Autodesk Fusion 360 part; units mm, degrees
(part 2 of 3)
sketch "Sketch7" plane through (0, 0, 3) normal (0, 0, 1) x (-1, 0, 0)
  line L0 (35, -173) -> (35, -178)
  line L1 (35, -178) -> (-35, -178)
  line L2 (-35, -178) -> (-35, -173)
  line L3 (-35, -173) -> (35, -173)
  line L4 (-35, -238) -> (-35, -233)
  line L5 (-35, -233) -> (35, -233)
  line L6 (35, -233) -> (35, -238)
  line L7 (35, -238) -> (-35, -238)
  circle A0 centre (-24.25, -133) radius 1.5
  circle A1 centre (24.25, -71.5) radius 1.5
  circle A2 centre (24.25, -133) radius 1.5
  circle A3 centre (-24.25, -71.5) radius 1.5
  line L8 (46.5, -10) -> (46.5, -15)
  line L9 (46.5, -15) -> (-46.5, -15)
  line L10 (-46.5, -15) -> (-46.5, -10)
  line L11 (-46.5, -10) -> (46.5, -10)
  line L12 (-46.5, -63) -> (-46.5, -58)
  line L13 (-46.5, -58) -> (46.5, -58)
  line L14 (46.5, -58) -> (46.5, -63)
  line L15 (46.5, -63) -> (-46.5, -63)
  line L16 (51.5, 0) -> (-51.5, 0)
  line L17 (-51.5, 0) -> (-51.5, -265)
  line L18 (-51.5, -265) -> (51.5, -265)
  line L19 (51.5, -265) -> (51.5, 0)
  line L20 (0, -238) -> (0, -248)
  line L21 (0, -248) -> (3, -248)
  line L22 (0, -248) -> (-3, -248)
  line L23 (0, -265) -> (0, -260)
  line L24 (3, -248) -> (3, -258)
  line L25 (3, -258) -> (8, -258)
  line L26 (3, -248) -> (8, -248)
  line L27 (8, -258) -> (8, -248)
  line L28 (-3, -248) -> (-3, -258)
  line L29 (-3, -258) -> (-8, -258)
  line L30 (-8, -258) -> (-8, -248)
  line L31 (-3, -248) -> (-8, -248)
  dimension "d38" = 10
  dimension "d39" = 3
  dimension "d40" = 3
  dimension "d41" = 5
  dimension "d42" = 10
  dimension "d43" = 5
  dimension "d44" = 5
  dimension "d45" = 5
  dimension "d46" = 10
  constraint midpoint L7 L20.start
  constraint perpendicular L7 L20
  constraint perpendicular L20 L21
  constraint perpendicular L20 L22
  constraint midpoint L18 L23.start
  constraint perpendicular L18 L23
  constraint perpendicular L21 L24
  constraint perpendicular L24 L25
  constraint perpendicular L20 L26
  constraint perpendicular L22 L28
  constraint perpendicular L28 L29
  constraint perpendicular L29 L30
  constraint perpendicular L30 L31
  measures "d38" distance of L20.start L20.end
  measures "d39" distance of L20.end L21.end
  measures "d40" distance of L20.end L22.end
  measures "d41" distance of L23.start L23.end
  measures "d42" distance of L21.end L24.end
  measures "d43" distance of L24.end L25.end
  measures "d44" distance of L21.end L26.end
  measures "d45" distance of L28.end L29.end
  measures "d46" distance of L29.end L30.end
extrude "Extrude7" add sketch "Sketch7" along normal blind 6 contours L24 L25 L26 L27 | L28 L29 L30 L31
sketch "Sketch8" plane through (8, 0, 0) normal (1, 0, 0) x (0, 1, 0)
  line L0 (248, 3) -> (258, 3)
  line L1 (258, 3) -> (258, 9)
  line L2 (258, 9) -> (248, 9)
  line L3 (248, 9) -> (248, 3)
  line L4 (253, 3) -> (253, 9)
  circle A0 centre (253, 6) radius 1.5
  dimension "d49" = 3
  constraint midpoint L0 L4.start
  constraint midpoint L2 L4.end
  constraint midpoint L4 A0.centre
  measures "d49" diameter of A0
extrude "Extrude8" cut sketch "Sketch8" against normal blind 20 contours L4 A0 | L4 A0
fillet "Fillet1" radius 10 4 edges at (51.5, 0, 1.5) (-51.5, 0, 1.5) (51.5, 265, 1.5) (-51.5, 265, 1.5)
fillet "Fillet2" radius 5 8 edges at (51.5, 132.5, 0) (48.5711, 262.0711, 0) (0, 265, 0) (-48.5711, 262.0711, 0) (-51.5, 132.5, 0) (-48.5711, 2.9289, 0) (0, 0, 0) (48.5711, 2.9289, 0)
sketch "Sketch9" plane through (0, 0, 3) normal (0, 0, 1) x (-1, 0, 0)
  arc A0 (41.5, -265) -> (51.5, -255) centre (41.5, -255) ccw
  line L0 (51.5, -255) -> (51.5, -10)
  arc A1 (51.5, -10) -> (41.5, 0) centre (41.5, -10) ccw
  line L1 (41.5, 0) -> (-41.5, 0)
  arc A2 (-41.5, 0) -> (-51.5, -10) centre (-41.5, -10) ccw
  line L2 (-51.5, -10) -> (-51.5, -255)
  arc A3 (-51.5, -255) -> (-41.5, -265) centre (-41.5, -255) ccw
  line L3 (-41.5, -265) -> (41.5, -265)
  line L4 (-3, -258) -> (-8, -258)
  line L5 (-8, -258) -> (-8, -248)
  line L6 (-8, -248) -> (-3, -248)
  line L7 (-3, -248) -> (-3, -258)
  line L8 (3, -248) -> (8, -248)
  line L9 (8, -248) -> (8, -258)
  line L10 (8, -258) -> (3, -258)
  line L11 (3, -258) -> (3, -248)
  line L12 (35, -173) -> (35, -178)
  line L13 (35, -178) -> (-35, -178)
  line L14 (-35, -178) -> (-35, -173)
  line L15 (-35, -173) -> (35, -173)
  line L16 (-35, -238) -> (-35, -233)
  line L17 (-35, -233) -> (35, -233)
  line L18 (35, -233) -> (35, -238)
  line L19 (35, -238) -> (-35, -238)
  circle A4 centre (-24.25, -133) radius 1.5
  circle A5 centre (24.25, -71.5) radius 1.5
  circle A6 centre (24.25, -133) radius 1.5
  circle A7 centre (-24.25, -71.5) radius 1.5
  line L20 (46.5, -10) -> (46.5, -15)
  line L21 (46.5, -15) -> (-46.5, -15)
  line L22 (-46.5, -15) -> (-46.5, -10)
  line L23 (-46.5, -10) -> (46.5, -10)
  line L24 (-46.5, -63) -> (-46.5, -58)
  line L25 (-46.5, -58) -> (46.5, -58)
  line L26 (46.5, -58) -> (46.5, -63)
  line L27 (46.5, -63) -> (-46.5, -63)
  line L28 (0, -58) -> (0, -15)
  line L29 (0, -36.5) -> (20, -36.5)
  line L30 (0, -36.5) -> (-20, -36.5)
  line L31 (20, -36.5) -> (20, -46.5)
  line L32 (-20, -36.5) -> (-20, -46.5)
  line L33 (20, -46.5) -> (-20, -46.5)
  line L34 (20, -36.5) -> (20, -26.5)
  line L35 (20, -26.5) -> (-20, -26.5)
  line L36 (-20, -36.5) -> (-20, -26.5)
  dimension "d56" = 20
  dimension "d57" = 20
  dimension "d58" = 10
  dimension "d59" = 10
  dimension "d60" = 10
  dimension "d61" = 40
  constraint midpoint L25 L28.start
  constraint midpoint L21 L28.end
  constraint midpoint L28 L29.start
  constraint perpendicular L28 L29
  constraint perpendicular L28 L30
  constraint perpendicular L25 L31
  constraint perpendicular L30 L32
  constraint perpendicular L29 L34
  constraint perpendicular L28 L35
  measures "d56" distance of L29.start L29.end
  measures "d57" distance of L29.start L30.end
  measures "d58" distance of L29.end L31.end
  measures "d59" distance of L30.end L32.end
  measures "d60" distance of L29.end L34.end
  measures "d61" distance of L34.end L35.end
extrude "Extrude9" cut sketch "Sketch9" against normal blind 5 contours L28 L30 L32 L33 | L28 L29 L31 L33 | L28 L30 L35 L36 | L28 L29 L34 L35
sketch "Sketch10" plane through (0, 0, 9) normal (0, 0, 1) x (-1, 0, 0)
  line L0 (-46.5, -63) -> (46.5, -63)
  line L1 (46.5, -63) -> (46.5, -58)
  line L2 (46.5, -58) -> (-46.5, -58)
  line L3 (-46.5, -58) -> (-46.5, -63)
  line L4 (46.5, -60.5) -> (28.5, -60.5)
  circle A0 centre (28.5, -60.5) radius 1.5
  line L5 (0, -58) -> (0, -50)
  line L6 (46.5, -58) -> (46.5, -15)
  line L7 (46.5, -36.5) -> (70, -36.5)
  circle A1 centre (28.5, -12.5) radius 1.5
  circle A2 centre (-28.5, -60.5) radius 1.5
  circle A3 centre (-28.5, -12.5) radius 1.5
  point P0 (28.5, -12.5)
  dimension "d64" = 18
  dimension "d65" = 3
  dimension "d66" = 3
  constraint midpoint L1 L4.start
  constraint perpendicular L1 L4
  constraint coincident L4.end A0.centre
  constraint midpoint L2 L5.start
  constraint perpendicular L2 L5
  constraint coincident L1.end L2.start
  constraint perpendicular L2 L6
  constraint midpoint L6 L7.start
  constraint perpendicular L6 L7
  constraint symmetric L4.end L7 P0
  constraint coincident P0 A1.centre
  constraint symmetric A0 L5 A2
  constraint symmetric L5 A1 A3
  measures "d64" distance of L4.start L4.end
  measures "d65" diameter of A0
  measures "d66" diameter of A1
extrude "Extrude10" cut sketch "Sketch10" against normal blind 50 contours A0 | A1 | A2 | A3
sketch "Sketch11" plane through (0, 0, 3) normal (0, 0, 1) x (-1, 0, 0)
  line L0 (-20, -26.5) -> (20, -26.5)
  line L1 (20, -26.5) -> (20, -46.5)
  line L2 (20, -46.5) -> (-20, -46.5)
  line L3 (-20, -46.5) -> (-20, -26.5)
  arc A0 (41.5, -265) -> (51.5, -255) centre (41.5, -255) ccw
  line L4 (51.5, -255) -> (51.5, -10)
  arc A1 (51.5, -10) -> (41.5, 0) centre (41.5, -10) ccw
  line L5 (41.5, 0) -> (-41.5, 0)
  arc A2 (-41.5, 0) -> (-51.5, -10) centre (-41.5, -10) ccw
  line L6 (-51.5, -10) -> (-51.5, -255)
  arc A3 (-51.5, -255) -> (-41.5, -265) centre (-41.5, -255) ccw
  line L7 (-41.5, -265) -> (41.5, -265)
  line L8 (-3, -258) -> (-8, -258)
  line L9 (-8, -258) -> (-8, -248)
  line L10 (-8, -248) -> (-3, -248)
  line L11 (-3, -248) -> (-3, -258)
  line L12 (3, -248) -> (8, -248)
  line L13 (8, -248) -> (8, -258)
  line L14 (8, -258) -> (3, -258)
  line L15 (3, -258) -> (3, -248)
  line L16 (35, -173) -> (35, -178)
  line L17 (35, -178) -> (-35, -178)
  line L18 (-35, -178) -> (-35, -173)
  line L19 (-35, -173) -> (35, -173)
  line L20 (-35, -238) -> (-35, -233)
  line L21 (-35, -233) -> (35, -233)
  line L22 (35, -233) -> (35, -238)
  line L23 (35, -238) -> (-35, -238)
  circle A4 centre (-24.25, -133) radius 1.5
  circle A5 centre (24.25, -71.5) radius 1.5
  circle A6 centre (24.25, -133) radius 1.5
  circle A7 centre (-24.25, -71.5) radius 1.5
  line L24 (46.5, -10) -> (46.5, -15)
  line L25 (46.5, -15) -> (-46.5, -15)
  line L26 (-46.5, -15) -> (-46.5, -10)
  line L27 (-46.5, -10) -> (46.5, -10)
  line L28 (-46.5, -63) -> (-46.5, -58)
  line L29 (-46.5, -58) -> (46.5, -58)
  line L30 (46.5, -58) -> (46.5, -63)
  line L31 (46.5, -63) -> (-46.5, -63)
  line L32 (51.5, -255) -> (48.5, -255)
  circle A8 centre (48.5, -255) radius 1.5
  line L33 (51.5, -132.5) -> (48.5, -132.5)
  circle A9 centre (48.5, -132.5) radius 1.5
  line L34 (48.5, -255) -> (48.5, -132.5)
  circle A10 centre (48.5, -193.75) radius 1.5
  line L35 (0, -265) -> (0, -262)
  circle A11 centre (0, -262) radius 1.5
  circle A12 centre (0, -3) radius 1.5
  circle A13 centre (48.5, -10) radius 1.5
  circle A14 centre (48.5, -71.25) radius 1.5
  circle A15 centre (48.5, -132.5) radius 1.5
  circle A16 centre (-48.5, -10) radius 1.5
  circle A17 centre (-48.5, -71.25) radius 1.5
  circle A18 centre (-48.5, -132.5) radius 1.5
  circle A19 centre (-48.5, -193.75) radius 1.5
  circle A20 centre (-48.5, -255) radius 1.5
  dimension "d69" = 3
  dimension "d70" = 3
  dimension "d71" = 3
  dimension "d72" = 3
  dimension "d73" = 3
  dimension "d74" = 3
  dimension "d75" = 3
  constraint coincident A0.end L4.start
  constraint perpendicular L4 L32
  constraint coincident L32.end A8.centre
  constraint midpoint L4 L33.start
  constraint perpendicular L4 L33
  constraint coincident L33.end A9.centre
  constraint midpoint L34 A10.centre
  constraint midpoint L7 L35.start
  constraint perpendicular L7 L35
  constraint coincident L35.end A11.centre
  constraint symmetric A8 L33 A13
  constraint symmetric L33 A9 A15
  constraint symmetric L33 A10 A14
  constraint symmetric L33 A11 A12
  constraint symmetric A8 L35 A20
  constraint symmetric A10 L35 A19
  constraint symmetric L35 A13 A16
  constraint symmetric L35 A14 A17
  constraint symmetric L35 A15 A18
  measures "d69" distance of A0.end L32.end
  measures "d70" diameter of A8
  measures "d71" distance of L33.start L33.end
  measures "d72" diameter of A9
  measures "d73" diameter of A10
  measures "d74" distance of L35.start L35.end
  measures "d75" diameter of A11
extrude "Extrude11" cut sketch "Sketch11" against normal blind 5 contours L32 A8 L34 | L32 A8 L34 | L33 A9 L34 A15 | L33 A9 L34 A15 | L34 A10 | L34 A10 | A11 | A12 | A13 | A14 | A16 | A17 | A18 | A19 | A20
sketch "Sketch12" plane through (0, 0, 3) normal (0, 0, 1) x (-1, 0, 0)
  circle A0 centre (48.5, -255) radius 1.5
  circle A1 centre (-48.5, -193.75) radius 1.5
  circle A2 centre (-48.5, -10) radius 1.5
  circle A3 centre (48.5, -10) radius 1.5
  circle A4 centre (-48.5, -132.5) radius 1.5
  circle A5 centre (0, -262) radius 1.5
  circle A6 centre (48.5, -193.75) radius 1.5
  circle A7 centre (-48.5, -71.25) radius 1.5
  circle A8 centre (0, -3) radius 1.5
  circle A9 centre (48.5, -71.25) radius 1.5
  circle A10 centre (48.5, -132.5) radius 1.5
  circle A11 centre (-48.5, -255) radius 1.5
  line L0 (-20, -26.5) -> (20, -26.5)
  line L1 (20, -26.5) -> (20, -46.5)
  line L2 (20, -46.5) -> (-20, -46.5)
  line L3 (-20, -46.5) -> (-20, -26.5)
  arc A12 (41.5, -265) -> (51.5, -255) centre (41.5, -255) ccw
  line L4 (51.5, -255) -> (51.5, -10)
  arc A13 (51.5, -10) -> (41.5, 0) centre (41.5, -10) ccw
  line L5 (41.5, 0) -> (-41.5, 0)
  arc A14 (-41.5, 0) -> (-51.5, -10) centre (-41.5, -10) ccw
  line L6 (-51.5, -10) -> (-51.5, -255)
  arc A15 (-51.5, -255) -> (-41.5, -265) centre (-41.5, -255) ccw
  line L7 (-41.5, -265) -> (41.5, -265)
  line L8 (-3, -258) -> (-8, -258)
  line L9 (-8, -258) -> (-8, -248)
  line L10 (-8, -248) -> (-3, -248)
  line L11 (-3, -248) -> (-3, -258)
  line L12 (3, -248) -> (8, -248)
  line L13 (8, -248) -> (8, -258)
  line L14 (8, -258) -> (3, -258)
  line L15 (3, -258) -> (3, -248)
  line L16 (35, -173) -> (35, -178)
  line L17 (35, -178) -> (-35, -178)
  line L18 (-35, -178) -> (-35, -173)
  line L19 (-35, -173) -> (35, -173)
  line L20 (-35, -238) -> (-35, -233)
  line L21 (-35, -233) -> (35, -233)
  line L22 (35, -233) -> (35, -238)
  line L23 (35, -238) -> (-35, -238)
  circle A16 centre (-24.25, -133) radius 1.5
  circle A17 centre (24.25, -71.5) radius 1.5
  circle A18 centre (24.25, -133) radius 1.5
  circle A19 centre (-24.25, -71.5) radius 1.5
  line L24 (46.5, -10) -> (46.5, -15)
  line L25 (46.5, -15) -> (-46.5, -15)
  line L26 (-46.5, -15) -> (-46.5, -10)
  line L27 (-46.5, -10) -> (46.5, -10)
  line L28 (-46.5, -63) -> (-46.5, -58)
  line L29 (-46.5, -58) -> (46.5, -58)
  line L30 (46.5, -58) -> (46.5, -63)
  line L31 (46.5, -63) -> (-46.5, -63)
  line L32 (0, -173) -> (0, -133)
  line L33 (0, -153) -> (51.5, -153)
  line L34 (0, -153) -> (-51.5, -153)
  line L35 (-51.5, -153) -> (-51.5, -280)
  line L36 (-51.5, -280) -> (51.5, -280)
  line L37 (51.5, -280) -> (51.5, -153)
  line L38 (-51.5, -153) -> (-51.5, 0)
  line L39 (-51.5, 0) -> (51.5, 0)
  line L40 (51.5, 0) -> (51.5, -153)
  constraint midpoint L19 L32.start
  constraint perpendicular L19 L32
  constraint midpoint L32 L33.start
  constraint coincident L4 L33.end
  constraint perpendicular L4 L33
  constraint coincident L6 L34.end
  constraint perpendicular L6 L34
  constraint perpendicular L34 L35
  constraint perpendicular L4 L36
  constraint perpendicular L33 L37
  constraint perpendicular L34 L38
  constraint perpendicular L4 L39
  constraint perpendicular L33 L40
sketch "Sketch16" plane through (0, 0, 9) normal (0, 0, 1) x (-1, 0, 0)
  circle A0 centre (-28.5, -12.5) radius 1.5
  circle A1 centre (28.5, -12.5) radius 1.5
  line L0 (46.5, -10) -> (-46.5, -10)
  line L1 (-46.5, -10) -> (-46.5, -15)
  line L2 (-46.5, -15) -> (46.5, -15)
  line L3 (46.5, -15) -> (46.5, -10)
  line L4 (46.5, -15) -> (40, -15)
  line L5 (40, -15) -> (40, -10)
  line L6 (40, -10) -> (46.5, -10)
  line L7 (46.5, -10) -> (46.5, -15)
  line L8 (-46.5, -15) -> (-40, -15)
  line L9 (-46.5, -10) -> (-40, -10)
  line L10 (-40, -10) -> (-40, -15)
  dimension "d82" = 6.5
  dimension "d83" = 6.5
  constraint coincident L2.end L3.start
  constraint perpendicular L3 L4
  constraint perpendicular L4 L5
  constraint coincident L0.start L3.end
  constraint perpendicular L3 L6
  constraint coincident L1.end L2.start
  constraint perpendicular L1 L8
  constraint coincident L0.end L1.start
  constraint coincident L0 L9.end
  constraint perpendicular L1 L9
  measures "d82" distance of L2.end L4.end
  measures "d83" distance of L1.end L8.end
extrude "Extrude13" cut sketch "Sketch16" against normal blind 6 contours L0 L2 L3 L4 L5 L6 L7 | L0 L1 L2 L8 L9 L10
extrude "Extrude12" cut sketch "Sketch12" along normal blind 10 and the other way blind 40 contours A12 L4 L6 A15 L7 L33 L34 L35 L37 | L8 L9 L10 L11 | L12 L13 L14 L15 | L16 L17 L18 L19 | L20 L21 L22 L23

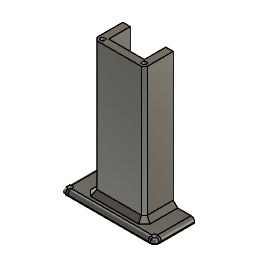
design "handlepiece2"
Autodesk Fusion 360 part; units mm, degrees
sketch "Sketch1" plane through (0, 0, 0) normal (0, 0, 1) x (1, 0, 0)
  line L0 (-28.5, -24) -> (-28.5, 24)
  line L1 (-28.5, 24) -> (28.5, 24)
  line L2 (28.5, 24) -> (28.5, -24)
  line L3 (-28.5, -24) -> (28.5, -24)
  circle A0 centre (-28.5, 24) radius 1.5
  circle A1 centre (28.5, 24) radius 1.5
  circle A2 centre (-28.5, -24) radius 1.5
  circle A3 centre (28.5, -24) radius 1.5
  line L4 (0, 24) -> (0, -24)
  line L5 (0, 0) -> (-28.5, 0)
  line L6 (-31.5, -27) -> (31.5, -27)
  line L7 (31.5, 27) -> (31.5, -27)
  line L8 (-31.5, 27) -> (31.5, 27)
  line L9 (-31.5, -27) -> (-31.5, 27)
  dimension "d1" = 3
  dimension "d2" = 3
  dimension "d3" = 3
  dimension "d4" = 3
  dimension "d5" = -3
  constraint perpendicular L0 L3
  constraint coincident L0.end L1.start
  constraint coincident L1.end L2.start
  constraint coincident L0.start L3.start
  constraint coincident L2.end L3.end
  constraint midpoint L1 L4.start
  constraint midpoint L3 L4.end
  constraint midpoint L4 L5.start
  constraint midpoint L0 L5.end
  constraint perpendicular L0 L5
  measures "d1" diameter of A0
  measures "d2" diameter of A1
  measures "d3" diameter of A2
  measures "d4" diameter of A3
extrude "Extrude1" add sketch "Sketch1" along normal blind 3 contours L0 L3 A2 L4 L5 | L0 L1 A0 L4 L5 | L1 L2 L3 A1 A3 L4 | L6 L7 L8 L9
sketch "Sketch2" plane through (0, 0, 3) normal (0, 0, 1) x (-1, 0, 0)
  circle A0 centre (-28.5, -24) radius 1.5
  circle A1 centre (28.5, 24) radius 1.5
  circle A2 centre (28.5, -24) radius 1.5
  circle A3 centre (-28.5, 24) radius 1.5
  line L0 (31.5, 27) -> (-31.5, 27)
  line L1 (-31.5, 27) -> (-31.5, -27)
  line L2 (-31.5, -27) -> (31.5, -27)
  line L3 (31.5, -27) -> (31.5, 27)
  line L4 (-15, -19.5) -> (15, -19.5)
  line L5 (12, -14.5) -> (-12, -14.5)
  circle A4 centre (14, -16.5) radius 1.5
  line L6 (15, -19.5) -> (17, -17.5)
  line L7 (17, -17.5) -> (17, 0)
  line L8 (17, 0) -> (12, 0)
  line L9 (12, 0) -> (12, -14.5)
  line L10 (-12, -14.5) -> (-12, 0)
  line L11 (-12, 0) -> (-17, 0)
  line L12 (-17, 0) -> (-17, -17.5)
  line L13 (-17, -17.5) -> (-15, -19.5)
  circle A5 centre (-14, -16.5) radius 1.5
  line L14 (12, 0) -> (-12, 0)
  line L15 (0, 0) -> (0, -7.25)
  line L16 (12, 0) -> (12, 14.5)
  line L17 (17, 17.5) -> (17, 0)
  line L18 (17, 0) -> (12, 0)
  line L19 (-15, 19.5) -> (15, 19.5)
  line L20 (12, 14.5) -> (-12, 14.5)
  line L21 (-12, 14.5) -> (-12, 0)
  circle A6 centre (14, 16.5) radius 1.5
  circle A7 centre (-14, 16.5) radius 1.5
  line L22 (-17, 17.5) -> (-15, 19.5)
  line L23 (-17, 0) -> (-17, 17.5)
  line L24 (-12, 0) -> (-17, 0)
  line L25 (15, 19.5) -> (17, 17.5)
  constraint perpendicular L10 L14
  constraint midpoint L14 L15.start
  constraint perpendicular L14 L15
  constraint symmetric L12.end L14 L22.start
  constraint symmetric L4.start L14 L19.start
  constraint symmetric L4.end L14 L19.end
  constraint symmetric L6.end L14 L17.start
  constraint symmetric L8.end L14 L9.start
  constraint symmetric L5.start L14 L16.end
  constraint symmetric L5.end L14 L20.end
  constraint symmetric L10.end L14 L11.start
  constraint symmetric L11.end L14 L12.start
  constraint symmetric L7.end L14 L8.start
  constraint symmetric A4 L14 A6
  constraint symmetric A5 L14 A7
extrude "Extrude2" add sketch "Sketch2" along normal blind 90 contours L4 L5 L6 L7 L8 L9 L10 L11 L12 L13 L18 L24 | L8 L11 L16 L17 L18 L19 L20 L21 L22 L23 L24 L25
fillet "Fillet1" radius 3 4 edges at (-31.5, -27, 1.5) (31.5, -27, 1.5) (31.5, 27, 1.5) (-31.5, 27, 1.5)
fillet "Fillet2" radius 2.5 8 edges at (30.6213, 26.1213, 3) (0, 27, 3) (-30.6213, 26.1213, 3) (-31.5, 0, 3) (-30.6213, -26.1213, 3) (0, -27, 3) (30.6213, -26.1213, 3) (31.5, 0, 3)
chamfer "Chamfer1" distance 3 angle 45 8 edges at (0, 19.5, 3) (17, 0, 3) (16, 18.5, 3) (-16, 18.5, 3) (-16, -18.5, 3) (-17, 0, 3) (0, -19.5, 3) (16, -18.5, 3)
sketch "Sketch3" plane through (0, 19.5, 0) normal (0, 1, 0) x (-1, 0, 0)
  line L0 (15, 6) -> (15, 93)
  line L1 (15, 93) -> (-15, 93)
  line L2 (-15, 93) -> (-15, 6)
  line L3 (-15, 49.5) -> (15, 49.5)
  circle A0 centre (0, 49.5) radius 9.5
  line L4 (-15, 6) -> (15, 6)
  dimension "d12" = 19
  constraint midpoint L2 L3.start
  constraint midpoint L0 L3.end
  constraint midpoint L3 A0.centre
  measures "d12" diameter of A0
extrude "Extrude3" cut sketch "Sketch3" against normal blind 6 contours L3 A0 | L3 A0
sketch "Sketch4" plane through (0, 0, 93) normal (0, 0, 1) x (-1, 0, 0)
  circle A0 centre (14, -16.5) radius 1.5
  circle A1 centre (14, 16.5) radius 1.5
  circle A2 centre (-14, -16.5) radius 1.5
  line L0 (12, 14.5) -> (12, -14.5)
  line L1 (12, -14.5) -> (-12, -14.5)
  line L2 (-12, -14.5) -> (-12, 14.5)
  line L3 (-12, 14.5) -> (12, 14.5)
  circle A3 centre (-14, 16.5) radius 1.5
  line L4 (-17, 17.5) -> (-17, -17.5)
  line L5 (-17, -17.5) -> (-15, -19.5)
  line L6 (-15, -19.5) -> (15, -19.5)
  line L7 (15, -19.5) -> (17, -17.5)
  line L8 (17, -17.5) -> (17, 17.5)
  line L9 (17, 17.5) -> (15, 19.5)
  line L10 (15, 19.5) -> (-15, 19.5)
  line L11 (-15, 19.5) -> (-17, 17.5)
  line L12 (-50, 0) -> (50, 0)
  line L13 (50, 0) -> (33.9234, 54.6299)
  line L14 (33.9234, 54.6299) -> (-46.2592, 44.9375)
  line L15 (-46.2592, 44.9375) -> (-50, 0)
  line L16 (12, 14.5) -> (-12, 14.5)
  line L17 (-12, 14.5) -> (-12, -14.5)
  line L18 (-12, -14.5) -> (12, -14.5)
  line L19 (12, -14.5) -> (12, 14.5)
  line L20 (-50, 0) -> (-64.2202, -68.1179)
  line L21 (-64.2202, -68.1179) -> (43.9074, -45.7813)
  line L22 (43.9074, -45.7813) -> (50, 0)
  constraint horizontal L12
extrude "Extrude4" cut sketch "Sketch4" against normal blind 500 contours A0 | A2 | L0 L2 L3 L12 L16 L17 L19 | L0 L1 L2 L4 L5 L6 L7 L8 L12 L17 L18 L19 | L0 L1 L2 L12 L17 L18 L19 | L4 L5 L6 L7 L8 L12 L20 L21 L22

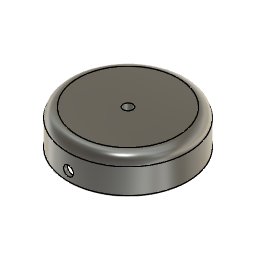
design "cap tesla coil"
Autodesk Fusion 360 part; units mm, degrees
sketch "Sketch1" plane through (0, 0, 0) normal (0, 0, 1) x (1, 0, 0)
  circle A0 centre (0, 0) radius 23
  circle A1 centre (0, 0) radius 24.5
  dimension "d1" = 46
  dimension "d2" = 49
  constraint coincident A0.centre A1.centre
  measures "d1" diameter of A0
  measures "d2" diameter of A1
extrude "Extrude1" add sketch "Sketch1" along normal blind 12
sketch "Sketch2" plane through (0, 0, 12) normal (0, 0, 1) x (-1, 0, 0)
  circle A0 centre (0, 0) radius 23
  circle A1 centre (0, 0) radius 24.5
  circle A2 centre (0, 0) radius 2
  circle A3 centre (0, 0) radius 24.5
  dimension "d5" = 4
  constraint coincident A0.centre A1.centre
  measures "d5" diameter of A2
extrude "Extrude2" add sketch "Sketch2" along normal blind 3 contours A0 | A1 A3
fillet "Fillet1" radius 4 1 edges at (22.842, 8.8596, 15)
sketch "Sketch3" plane through (0, 0, 0) normal (0, 1, 0) x (1, 0, 0)
  line L0 (0, 0) -> (0, -4.5)
  circle A0 centre (0, -4.5) radius 2
  dimension "d10" = 4.5
  dimension "d11" = 4
  constraint coincident L0.start origin
  constraint vertical L0
  constraint coincident L0.end A0.centre
  measures "d10" distance of L0.start L0.end
  measures "d11" diameter of A0
extrude "Extrude3" cut sketch "Sketch3" along normal mid plane 700
fillet "Fillet2" radius 0.75 2 edges at (-22.842, -8.8596, 0) (-21.4435, 8.3172, 0)

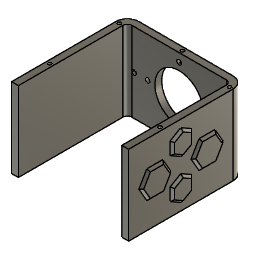
design "walls2"
Autodesk Fusion 360 part; units mm, degrees
sketch "Sketch1" plane through (0, 0, 0) normal (0, 0, 1) x (1, 0, 0)
  line L0 (41.5, 125) -> (-41.5, 125)
  arc A0 (-41.5, 125) -> (-51.5, 115) centre (-41.5, 115) ccw
  line L1 (-51.5, 115) -> (-51.5, -130)
  arc A1 (51.5, 115) -> (41.5, 125) centre (41.5, 115) ccw
  line L2 (51.5, -130) -> (51.5, 115)
  line L3 (-41.5, -140) -> (41.5, -140)
  arc A2 (41.5, -140) -> (51.5, -130) centre (41.5, -130) ccw
  arc A3 (-51.5, -130) -> (-41.5, -140) centre (-41.5, -130) ccw
  line L4 (0, 125) -> (0, 122)
  line L5 (-51.5, 115) -> (-48.5, 115)
  circle A4 centre (-48.5, 115) radius 1.5
  circle A5 centre (0, 122) radius 1.5
  circle A6 centre (-48.5, -7.5) radius 1.5
  circle A7 centre (-48.5, 53.75) radius 1.5
  circle A8 centre (-48.5, -130) radius 1.5
  circle A9 centre (-48.5, -68.75) radius 1.5
  circle A10 centre (-48.5, -7.5) radius 1.5
  circle A11 centre (48.5, 115) radius 1.5
  circle A12 centre (48.5, 53.75) radius 1.5
  circle A13 centre (48.5, -7.5) radius 1.5
  circle A14 centre (48.5, -68.75) radius 1.5
  circle A15 centre (48.5, -130) radius 1.5
  line L6 (0, -140) -> (0, -137)
  circle A16 centre (0, -137) radius 1.5
  arc A17 (-45.5, -130) -> (-41.5, -134) centre (-41.5, -130) ccw
  line L7 (-41.5, -134) -> (41.5, -134)
  arc A18 (41.5, -134) -> (45.5, -130) centre (41.5, -130) ccw
  arc A19 (45.5, 115) -> (41.5, 119) centre (41.5, 115) ccw
  line L8 (41.5, 119) -> (-41.5, 119)
  line L9 (-48.5, -99.375) -> (-48.5, -75)
  line L10 (-48.5, -99.375) -> (-48.5, -125)
  line L11 (-45.5, 115) -> (-45.5, -75)
  line L12 (-45.5, -125) -> (-45.5, -130)
  line L13 (45.5, -130) -> (45.5, -125)
  line L14 (45.5, -75) -> (45.5, 115)
  line L15 (-48.5, -75) -> (-45.5, -75)
  line L16 (45.5, -75) -> (48.5, -75)
  line L17 (-48.5, -125) -> (-45.5, -125)
  line L18 (45.5, -125) -> (48.5, -125)
  line L19 (-48.5, -75) -> (-48.5, -125)
  line L20 (48.5, -75) -> (48.5, -125)
  arc A20 (-41.5, 119) -> (-45.5, 115) centre (-41.5, 115) ccw
  dimension "d1" = 3
  dimension "d3" = 3
  dimension "d4" = 3
  dimension "d5" = 3
  dimension "d7" = 3
  dimension "d8" = 3
  dimension "d9" = 3
  dimension "d10" = 3
  constraint midpoint L0 L4.start
  constraint perpendicular L0 L4
  constraint coincident L5.end A4.centre
  constraint coincident L4.end A5.centre
  constraint symmetric L4 A4 A11
  constraint symmetric L4 A7 A12
  constraint symmetric L4 A8 A15
  constraint symmetric L4 A9 A14
  constraint symmetric L4 A10 A13
  constraint midpoint L3 L6.start
  constraint perpendicular L3 L6
  constraint coincident L6.end A16.centre
  constraint perpendicular L10 L15
  constraint concentric A3 A17
  constraint concentric A2 A18
  constraint concentric A1 A19
  constraint tangent L7 A18
  constraint tangent A17 L7
  constraint tangent A17 L11
  constraint tangent A19 L13
  constraint tangent A18 L13
  constraint tangent A19 L8
  constraint collinear L11 L12
  constraint coincident L13.end L17
  constraint coincident L14.start L15
  constraint collinear L13 L14
  constraint collinear L15 L16
  constraint collinear L17 L18
  constraint symmetric L4 A19.start L11.start
  constraint symmetric L4 A19.end L8.end
  constraint symmetric L4 A19 A20
  measures "d1" distance of L4.start L4.end
  measures "d3" distance of A0.end L5.end
  measures "d4" diameter of A4
  measures "d5" diameter of A5
  measures "d7" diameter of A6
  measures "d8" diameter of A7
  measures "d9" distance of L6.start L6.end
  measures "d10" diameter of A16
extrude "Extrude1" add sketch "Sketch1" along normal blind 70
fillet "Fillet1" radius 5 4 edges at (45.5, -125, 35) (45.5, -75, 35) (-45.5, -75, 35) (-45.5, -125, 35)
sketch "Sketch2" plane through (0, 0, 70) normal (0, 0, 1) x (-1, 0, 0)
  arc A0 (45.5, 129.5826) -> (48.5, 125) centre (50.5, 129.5826) ccw
  line L0 (48.5, 125) -> (48.5, 75)
  arc A1 (48.5, 75) -> (45.5, 70.4174) centre (50.5, 70.4174) ccw
  line L1 (45.5, 70.4174) -> (45.5, -115)
  arc A2 (41.5, -119) -> (45.5, -115) centre (41.5, -115) ccw
  line L2 (41.5, -119) -> (-41.5, -119)
  arc A3 (-45.5, -115) -> (-41.5, -119) centre (-41.5, -115) ccw
  line L3 (-45.5, -115) -> (-45.5, 70.4174)
  arc A4 (-45.5, 70.4174) -> (-48.5, 75) centre (-50.5, 70.4174) ccw
  line L4 (-48.5, 75) -> (-48.5, 125)
  arc A5 (-48.5, 125) -> (-45.5, 129.5826) centre (-50.5, 129.5826) ccw
  line L5 (-45.5, 129.5826) -> (-45.5, 130)
  arc A6 (-41.5, 134) -> (-45.5, 130) centre (-41.5, 130) ccw
  line L6 (-41.5, 134) -> (41.5, 134)
  arc A7 (45.5, 130) -> (41.5, 134) centre (41.5, 130) ccw
  line L7 (45.5, 130) -> (45.5, 129.5826)
  circle A8 centre (48.5, -115) radius 1.5
  circle A9 centre (0, 137) radius 1.5
  circle A10 centre (0, -122) radius 1.5
  circle A11 centre (-48.5, 68.75) radius 1.5
  circle A12 centre (48.5, 130) radius 1.5
  circle A13 centre (-48.5, -115) radius 1.5
  circle A14 centre (-48.5, 130) radius 1.5
  circle A15 centre (48.5, 7.5) radius 1.5
  circle A16 centre (48.5, -53.75) radius 1.5
  circle A17 centre (-48.5, -53.75) radius 1.5
  circle A18 centre (-48.5, 7.5) radius 1.5
  circle A19 centre (48.5, 68.75) radius 1.5
  arc A20 (51.5, 130) -> (41.5, 140) centre (41.5, 130) ccw
  line L8 (41.5, 140) -> (-41.5, 140)
  arc A21 (-41.5, 140) -> (-51.5, 130) centre (-41.5, 130) ccw
  line L9 (-51.5, 130) -> (-51.5, -115)
  arc A22 (-51.5, -115) -> (-41.5, -125) centre (-41.5, -115) ccw
  line L10 (-41.5, -125) -> (41.5, -125)
  arc A23 (41.5, -125) -> (51.5, -115) centre (41.5, -115) ccw
  line L11 (51.5, -115) -> (51.5, 130)
  line L12 (48.5, -53.75) -> (48.5, 7.5)
  line L13 (-48.5, -53.75) -> (-48.5, 7.5)
  line L14 (48.5, -23.125) -> (-48.5, -23.125)
  line L15 (51.5, -23.125) -> (48.5, -23.125)
  line L16 (-48.5, -23.125) -> (-56, -23.125)
  constraint coincident A16.centre L12.start
  constraint coincident A15.centre L12.end
  constraint coincident A17.centre L13.start
  constraint coincident A18.centre L13.end
  constraint midpoint L12 L14.start
  constraint midpoint L13 L14.end
  constraint coincident L11 L15.start
  constraint perpendicular L12 L15
  constraint perpendicular L9 L16
extrude "Extrude2" cut sketch "Sketch2" against normal blind 80 contours A0 L0 A1 L1 L3 A4 L4 A5 L5 A6 L6 A7 L7 A20 L8 A21 L9 L11 L14 L15 L16
sketch "Sketch3" plane through (0, 125, 0) normal (0, 1, 0) x (-1, 0, 0)
  line L0 (-41.5, 0) -> (41.5, 0)
  line L1 (41.5, 0) -> (41.5, 70)
  line L2 (41.5, 70) -> (-41.5, 70)
  line L3 (-41.5, 70) -> (-41.5, 0)
  line L4 (0, 70) -> (0, 0)
  line L5 (0, 35) -> (-16.6685, 35)
  line L6 (2, 37) -> (2, 56.1557)
  arc A0 (2, 13.8443) -> (21.1557, 33) centre (0, 35) ccw
  arc A1 (-2, 56.1557) -> (-21.1557, 37) centre (0, 35) ccw
  line L7 (21.1557, 37) -> (2, 37)
  line L8 (-2, 33) -> (-2, 13.8443)
  line L9 (2, 33) -> (21.1557, 33)
  line L10 (-21.1557, 33) -> (-2, 33)
  circle A2 centre (0, 35) radius 32.5
  line L11 (-2, 37) -> (-21.1557, 37)
  circle A3 centre (0, 7.375) radius 2
  arc A4 (-21.1557, 33) -> (-2, 13.8443) centre (0, 35) ccw
  circle A5 centre (0, 62.625) radius 2
  line L12 (-2, 56.1557) -> (-2, 37)
  line L13 (2, 13.8443) -> (2, 33)
  circle A6 centre (27.625, 35) radius 2
  circle A7 centre (-27.625, 35) radius 2
  arc A8 (21.1557, 37) -> (2, 56.1557) centre (0, 35) ccw
  line L14 (-27.625, 35) -> (-39.625, 35)
  circle A9 centre (-39.625, 35) radius 2
  line L15 (27.625, 35) -> (39.625, 35)
  circle A10 centre (39.625, 35) radius 2
  circle A11 centre (0, 35) radius 21.25
  point P0 (0, 35)
  dimension "d18" = 12
  dimension "d19" = 4
  dimension "d20" = 12
  dimension "d21" = 4
  constraint midpoint L2 L4.start
  constraint coincident L4.end origin
  constraint midpoint L4 P0
  constraint perpendicular L4 L5
  constraint coincident A7.centre L14.start
  constraint perpendicular L3 L14
  constraint coincident L14.end A9.centre
  constraint coincident A6.centre L15.start
  constraint horizontal L15
  constraint coincident L15.end A10.centre
  constraint coincident P0 L5.start
  measures "d18" distance of A7.centre L14.end
  measures "d19" diameter of A9
  measures "d20" distance of A6.centre L15.end
  measures "d21" diameter of A10
extrude "Extrude3" cut sketch "Sketch3" against normal blind 10 contours L3 A9 | L1 A10 | L4 A3 | L4 A3 | L4 L8 L10 L11 L12 A11 | L4 L6 L7 L9 L13 A11 | L4 A5 | L4 A5 | L8 L10 A4 A11 | A0 L9 L13 A11 | L6 L7 A8 A11 | A1 L11 L12 A11 | A6 | A7 picked at (-40.0166, 34.7473) picked at (40.429, 35.5515)
sketch "Sketch4" plane through (51.5, 0, 0) normal (1, 0, 0) x (0, 1, 0)
  line L0 (23.125, 70) -> (23.125, 0)
  line L1 (23.125, 0) -> (115, 0)
  line L2 (115, 0) -> (115, 70)
  line L3 (115, 70) -> (23.125, 70)
  line L4 (69.0625, 70) -> (69.0625, 0)
  line L5 (23.125, 35) -> (69.0625, 35)
  line L6 (69.0625, 70) -> (69.0625, 35)
  line L7 (69.0625, 41.5) -> (78.5888, 47)
  line L8 (78.5888, 47) -> (78.5888, 58)
  line L9 (78.5888, 58) -> (69.0625, 63.5)
  line L10 (69.0625, 63.5) -> (59.5362, 58)
  line L11 (59.5362, 58) -> (59.5362, 47)
  line L12 (59.5362, 47) -> (69.0625, 41.5)
  line L13 (59.5362, 12) -> (59.5362, 23)
  line L14 (69.0625, 6.5) -> (59.5362, 12)
  line L15 (78.5888, 12) -> (69.0625, 6.5)
  line L16 (78.5888, 23) -> (78.5888, 12)
  line L17 (69.0625, 28.5) -> (78.5888, 23)
  line L18 (59.5362, 23) -> (69.0625, 28.5)
  line L19 (32.0937, 35) -> (39.0937, 22.8756)
  line L20 (39.0937, 22.8756) -> (53.0937, 22.8756)
  line L21 (53.0937, 22.8756) -> (60.0937, 35)
  line L22 (60.0937, 35) -> (53.0937, 47.1244)
  line L23 (53.0937, 47.1244) -> (39.0937, 47.1244)
  line L24 (39.0937, 47.1244) -> (32.0937, 35)
  line L25 (85.0312, 47.1244) -> (99.0312, 47.1244)
  line L26 (99.0312, 47.1244) -> (106.0312, 35)
  line L27 (106.0312, 35) -> (99.0312, 22.8756)
  line L28 (99.0312, 22.8756) -> (85.0312, 22.8756)
  line L29 (85.0312, 22.8756) -> (78.0312, 35)
  line L30 (78.0312, 35) -> (85.0312, 47.1244)
  point P0 (69.0625, 52.5)
  point P1 (46.0937, 35)
  dimension "d24" = 11
  dimension "d25" = 14
  constraint midpoint L3 L4.start
  constraint midpoint L1 L4.end
  constraint midpoint L0 L5.start
  constraint midpoint L4 L5.end
  constraint midpoint L6 P0
  constraint symmetric L5 L7.start L17.start
  constraint symmetric L5 L7.end L16.start
  constraint symmetric L5 L8.end L15.start
  constraint symmetric L5 L9.end L14.start
  constraint symmetric L5 L10.end L13.start
  constraint symmetric L5 L11.end L13.end
  constraint midpoint L5 P1
  constraint symmetric L6 L19.start L26.end
  constraint symmetric L6 L19.end L27.end
  constraint symmetric L6 L20.end L28.end
  constraint symmetric L6 L21.end L29.end
  constraint symmetric L6 L22.end L25.start
  constraint symmetric L6 L23.end L25.end
  measures "d24" distance of L7.start P0
  measures "d25" distance of L19.start P1
extrude "Extrude4" add sketch "Sketch4" along normal blind 2 contours L5 L22 L23 L24 | L5 L19 L20 L21 | L4 L6 L7 L8 L9 | L4 L6 L10 L11 L12 | L4 L13 L14 L18 | L4 L15 L16 L17 | L25 L26 L27 L28 L29 L30
chamfer "Chamfer1" distance 2 angle 45 24 edges at (53.5, 46.0937, 47.1244) (53.5, 35.5937, 41.0622) (53.5, 35.5937, 28.9378) (53.5, 56.5937, 41.0622) (53.5, 81.5312, 41.0622) (53.5, 92.0312, 47.1244) (53.5, 102.5312, 41.0622) (53.5, 102.5312, 28.9378) (53.5, 92.0312, 22.8756) (53.5, 81.5312, 28.9378) (53.5, 56.5937, 28.9378) (53.5, 46.0937, 22.8756) (53.5, 64.2994, 25.75) (53.5, 73.8256, 25.75) (53.5, 78.5888, 17.5) (53.5, 73.8256, 9.25) (53.5, 64.2994, 9.25) (53.5, 59.5362, 17.5) (53.5, 64.2994, 60.75) (53.5, 73.8256, 60.75) (53.5, 78.5888, 52.5) (53.5, 73.8256, 44.25) (53.5, 64.2994, 44.25) (53.5, 59.5362, 52.5)
sketch "Sketch6" plane through (-51.5, 0, 0) normal (-1, 0, 0) x (0, -1, 0)
  line L0 (-23.125, 0) -> (-23.125, 70)
  line L1 (-23.125, 70) -> (-115, 70)
  line L2 (-115, 70) -> (-115, 0)
  line L3 (-115, 0) -> (-23.125, 0)
  line L4 (-59.5362, 47) -> (-69.0625, 41.5)
  line L5 (-69.0625, 41.5) -> (-78.5888, 47)
  line L6 (-78.5888, 47) -> (-78.5888, 58)
  line L7 (-78.5888, 58) -> (-69.0625, 63.5)
  line L8 (-69.0625, 63.5) -> (-59.5362, 58)
  line L9 (-59.5362, 58) -> (-59.5362, 47)
  line L10 (-60.0937, 35) -> (-53.0937, 47.1244)
  line L11 (-53.0937, 47.1244) -> (-39.0937, 47.1244)
  line L12 (-39.0937, 47.1244) -> (-32.0937, 35)
  line L13 (-32.0937, 35) -> (-39.0937, 22.8756)
  line L14 (-39.0937, 22.8756) -> (-53.0937, 22.8756)
  line L15 (-53.0937, 22.8756) -> (-60.0937, 35)
  line L16 (-59.5362, 23) -> (-69.0625, 28.5)
  line L17 (-59.5362, 12) -> (-59.5362, 23)
  line L18 (-69.0625, 6.5) -> (-59.5362, 12)
  line L19 (-78.5888, 12) -> (-69.0625, 6.5)
  line L20 (-78.5888, 23) -> (-78.5888, 12)
  line L21 (-69.0625, 28.5) -> (-78.5888, 23)
  line L22 (-99.0312, 22.8756) -> (-85.0312, 22.8756)
  line L23 (-78.0312, 35) -> (-85.0312, 47.1244)
  line L24 (-85.0312, 22.8756) -> (-78.0312, 35)
  line L25 (-85.0312, 47.1244) -> (-99.0312, 47.1244)
  line L26 (-99.0312, 47.1244) -> (-106.0312, 35)
  line L27 (-106.0312, 35) -> (-99.0312, 22.8756)
extrude "Extrude5" add sketch "Sketch6" along normal blind 2 contours L4 L5 L6 L7 L8 L9 | L10 L11 L12 L13 L14 L15 | L16 L17 L18 L19 L20 L21 | L22 L23 L24 L25 L26 L27
chamfer "Chamfer2" distance 2 angle 45 24 edges at (-53.5, 73.8256, 60.75) (-53.5, 64.2994, 60.75) (-53.5, 59.5362, 52.5) (-53.5, 64.2994, 44.25) (-53.5, 73.8256, 44.25) (-53.5, 78.5888, 52.5) (-53.5, 92.0312, 47.1244) (-53.5, 81.5312, 41.0622) (-53.5, 81.5312, 28.9378) (-53.5, 92.0312, 22.8756) (-53.5, 102.5312, 28.9378) (-53.5, 102.5312, 41.0622) (-53.5, 73.8256, 25.75) (-53.5, 64.2994, 25.75) (-53.5, 59.5362, 17.5) (-53.5, 64.2994, 9.25) (-53.5, 73.8256, 9.25) (-53.5, 78.5888, 17.5) (-53.5, 56.5937, 41.0622) (-53.5, 46.0937, 47.1244) (-53.5, 35.5937, 41.0622) (-53.5, 35.5937, 28.9378) (-53.5, 46.0937, 22.8756) (-53.5, 56.5937, 28.9378)

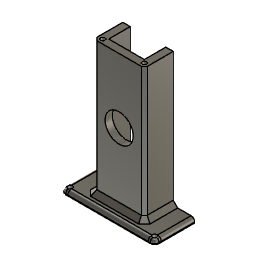
design "handlepiece1"
Autodesk Fusion 360 part; units mm, degrees
sketch "Sketch1" plane through (0, 0, 0) normal (0, 0, 1) x (1, 0, 0)
  line L0 (-28.5, -24) -> (-28.5, 24)
  line L1 (-28.5, 24) -> (28.5, 24)
  line L2 (28.5, 24) -> (28.5, -24)
  line L3 (-28.5, -24) -> (28.5, -24)
  circle A0 centre (-28.5, 24) radius 1.5
  circle A1 centre (28.5, 24) radius 1.5
  circle A2 centre (-28.5, -24) radius 1.5
  circle A3 centre (28.5, -24) radius 1.5
  line L4 (0, 24) -> (0, -24)
  line L5 (0, 0) -> (-28.5, 0)
  line L6 (-31.5, -27) -> (31.5, -27)
  line L7 (31.5, 27) -> (31.5, -27)
  line L8 (-31.5, 27) -> (31.5, 27)
  line L9 (-31.5, -27) -> (-31.5, 27)
  dimension "d1" = 3
  dimension "d2" = 3
  dimension "d3" = 3
  dimension "d4" = 3
  dimension "d5" = -3
  constraint perpendicular L0 L3
  constraint coincident L0.end L1.start
  constraint coincident L1.end L2.start
  constraint coincident L0.start L3.start
  constraint coincident L2.end L3.end
  constraint midpoint L1 L4.start
  constraint midpoint L3 L4.end
  constraint midpoint L4 L5.start
  constraint midpoint L0 L5.end
  constraint perpendicular L0 L5
  measures "d1" diameter of A0
  measures "d2" diameter of A1
  measures "d3" diameter of A2
  measures "d4" diameter of A3
extrude "Extrude1" add sketch "Sketch1" along normal blind 3 contours L0 L3 A2 L4 L5 | L0 L1 A0 L4 L5 | L1 L2 L3 A1 A3 L4 | L6 L7 L8 L9
sketch "Sketch2" plane through (0, 0, 3) normal (0, 0, 1) x (-1, 0, 0)
  circle A0 centre (-28.5, -24) radius 1.5
  circle A1 centre (28.5, 24) radius 1.5
  circle A2 centre (28.5, -24) radius 1.5
  circle A3 centre (-28.5, 24) radius 1.5
  line L0 (31.5, 27) -> (-31.5, 27)
  line L1 (-31.5, 27) -> (-31.5, -27)
  line L2 (-31.5, -27) -> (31.5, -27)
  line L3 (31.5, -27) -> (31.5, 27)
  line L4 (-15, -19.5) -> (15, -19.5)
  line L5 (12, -14.5) -> (-12, -14.5)
  circle A4 centre (14, -16.5) radius 1.5
  line L6 (15, -19.5) -> (17, -17.5)
  line L7 (17, -17.5) -> (17, 0)
  line L8 (17, 0) -> (12, 0)
  line L9 (12, 0) -> (12, -14.5)
  line L10 (-12, -14.5) -> (-12, 0)
  line L11 (-12, 0) -> (-17, 0)
  line L12 (-17, 0) -> (-17, -17.5)
  line L13 (-17, -17.5) -> (-15, -19.5)
  circle A5 centre (-14, -16.5) radius 1.5
  line L14 (12, 0) -> (-12, 0)
  line L15 (0, 0) -> (0, -7.25)
  line L16 (12, 0) -> (12, 14.5)
  line L17 (17, 17.5) -> (17, 0)
  line L18 (17, 0) -> (12, 0)
  line L19 (-15, 19.5) -> (15, 19.5)
  line L20 (12, 14.5) -> (-12, 14.5)
  line L21 (-12, 14.5) -> (-12, 0)
  circle A6 centre (14, 16.5) radius 1.5
  circle A7 centre (-14, 16.5) radius 1.5
  line L22 (-17, 17.5) -> (-15, 19.5)
  line L23 (-17, 0) -> (-17, 17.5)
  line L24 (-12, 0) -> (-17, 0)
  line L25 (15, 19.5) -> (17, 17.5)
  constraint perpendicular L10 L14
  constraint midpoint L14 L15.start
  constraint perpendicular L14 L15
  constraint symmetric L12.end L14 L22.start
  constraint symmetric L4.start L14 L19.start
  constraint symmetric L4.end L14 L19.end
  constraint symmetric L6.end L14 L17.start
  constraint symmetric L8.end L14 L9.start
  constraint symmetric L5.start L14 L16.end
  constraint symmetric L5.end L14 L20.end
  constraint symmetric L10.end L14 L11.start
  constraint symmetric L11.end L14 L12.start
  constraint symmetric L7.end L14 L8.start
  constraint symmetric A4 L14 A6
  constraint symmetric A5 L14 A7
extrude "Extrude2" add sketch "Sketch2" along normal blind 90 contours L4 L5 L6 L7 L8 L9 L10 L11 L12 L13 L18 L24 | L8 L11 L16 L17 L18 L19 L20 L21 L22 L23 L24 L25
fillet "Fillet1" radius 3 4 edges at (-31.5, -27, 1.5) (31.5, -27, 1.5) (31.5, 27, 1.5) (-31.5, 27, 1.5)
fillet "Fillet2" radius 2.5 8 edges at (30.6213, 26.1213, 3) (0, 27, 3) (-30.6213, 26.1213, 3) (-31.5, 0, 3) (-30.6213, -26.1213, 3) (0, -27, 3) (30.6213, -26.1213, 3) (31.5, 0, 3)
chamfer "Chamfer1" distance 3 angle 45 8 edges at (0, 19.5, 3) (17, 0, 3) (16, 18.5, 3) (-16, 18.5, 3) (-16, -18.5, 3) (-17, 0, 3) (0, -19.5, 3) (16, -18.5, 3)
sketch "Sketch3" plane through (0, 19.5, 0) normal (0, 1, 0) x (-1, 0, 0)
  line L0 (15, 6) -> (15, 93)
  line L1 (15, 93) -> (-15, 93)
  line L2 (-15, 93) -> (-15, 6)
  line L3 (-15, 49.5) -> (15, 49.5)
  circle A0 centre (0, 49.5) radius 9.5
  line L4 (-15, 6) -> (15, 6)
  dimension "d12" = 19
  constraint midpoint L2 L3.start
  constraint midpoint L0 L3.end
  constraint midpoint L3 A0.centre
  measures "d12" diameter of A0
extrude "Extrude3" cut sketch "Sketch3" against normal blind 6 contours L3 A0 | L3 A0
sketch "Sketch4" plane through (0, 0, 93) normal (0, 0, 1) x (-1, 0, 0)
  circle A0 centre (14, -16.5) radius 1.5
  circle A1 centre (14, 16.5) radius 1.5
  circle A2 centre (-14, -16.5) radius 1.5
  line L0 (12, 14.5) -> (12, -14.5)
  line L1 (12, -14.5) -> (-12, -14.5)
  line L2 (-12, -14.5) -> (-12, 14.5)
  line L3 (-12, 14.5) -> (12, 14.5)
  circle A3 centre (-14, 16.5) radius 1.5
  line L4 (-17, 17.5) -> (-17, -17.5)
  line L5 (-17, -17.5) -> (-15, -19.5)
  line L6 (-15, -19.5) -> (15, -19.5)
  line L7 (15, -19.5) -> (17, -17.5)
  line L8 (17, -17.5) -> (17, 17.5)
  line L9 (17, 17.5) -> (15, 19.5)
  line L10 (15, 19.5) -> (-15, 19.5)
  line L11 (-15, 19.5) -> (-17, 17.5)
  line L12 (-50, 0) -> (50, 0)
  line L13 (50, 0) -> (33.9234, 54.6299)
  line L14 (33.9234, 54.6299) -> (-46.2592, 44.9375)
  line L15 (-46.2592, 44.9375) -> (-50, 0)
  line L16 (12, 14.5) -> (-12, 14.5)
  line L17 (-12, 14.5) -> (-12, -14.5)
  line L18 (-12, -14.5) -> (12, -14.5)
  line L19 (12, -14.5) -> (12, 14.5)
  line L20 (-50, 0) -> (-64.2202, -68.1179)
  line L21 (-64.2202, -68.1179) -> (43.9074, -45.7813)
  line L22 (43.9074, -45.7813) -> (50, 0)
  constraint horizontal L12
extrude "Extrude4" cut sketch "Sketch4" against normal blind 500 contours A0 | A2 | L0 L2 L3 L12 L16 L17 L19 | L0 L1 L2 L4 L5 L6 L7 L8 L12 L17 L18 L19 | L0 L1 L2 L12 L17 L18 L19 | L4 L5 L6 L7 L8 L12 L20 L21 L22
sketch "Sketch5" plane through (0, -19.5, 0) normal (0, -1, 0) x (1, 0, 0)
  line L0 (-15, 6) -> (15, 6)
  line L1 (15, 6) -> (15, 93)
  line L2 (15, 93) -> (-15, 93)
  line L3 (-15, 93) -> (-15, 6)
  line L4 (-15, 49.5) -> (15, 49.5)
  circle A0 centre (0, 49.5) radius 9.5
  dimension "d22" = 19
  constraint midpoint L3 L4.start
  constraint midpoint L1 L4.end
  constraint midpoint L4 A0.centre
  measures "d22" diameter of A0
extrude "Extrude5" cut sketch "Sketch5" against normal blind 10 contours L4 A0 | L4 A0

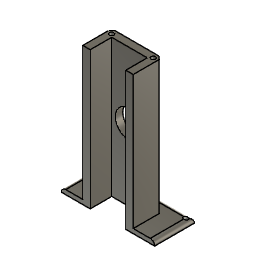
design "handlepiece1"
Autodesk Fusion 360 part; units mm, degrees
sketch "Sketch1" plane through (0, 0, 0) normal (0, 0, 1) x (1, 0, 0)
  line L0 (-28.5, -24) -> (-28.5, 24)
  line L1 (-28.5, 24) -> (28.5, 24)
  line L2 (28.5, 24) -> (28.5, -24)
  line L3 (-28.5, -24) -> (28.5, -24)
  circle A0 centre (-28.5, 24) radius 1.5
  circle A1 centre (28.5, 24) radius 1.5
  circle A2 centre (-28.5, -24) radius 1.5
  circle A3 centre (28.5, -24) radius 1.5
  line L4 (0, 24) -> (0, -24)
  line L5 (0, 0) -> (-28.5, 0)
  line L6 (-31.5, -27) -> (31.5, -27)
  line L7 (31.5, 27) -> (31.5, -27)
  line L8 (-31.5, 27) -> (31.5, 27)
  line L9 (-31.5, -27) -> (-31.5, 27)
  dimension "d1" = 3
  dimension "d2" = 3
  dimension "d3" = 3
  dimension "d4" = 3
  dimension "d5" = -3
  constraint perpendicular L0 L3
  constraint coincident L0.end L1.start
  constraint coincident L1.end L2.start
  constraint coincident L0.start L3.start
  constraint coincident L2.end L3.end
  constraint midpoint L1 L4.start
  constraint midpoint L3 L4.end
  constraint midpoint L4 L5.start
  constraint midpoint L0 L5.end
  constraint perpendicular L0 L5
  measures "d1" diameter of A0
  measures "d2" diameter of A1
  measures "d3" diameter of A2
  measures "d4" diameter of A3
extrude "Extrude1" add sketch "Sketch1" along normal blind 3 contours L0 L3 A2 L4 L5 | L0 L1 A0 L4 L5 | L1 L2 L3 A1 A3 L4 | L6 L7 L8 L9
sketch "Sketch2" plane through (0, 0, 3) normal (0, 0, 1) x (-1, 0, 0)
  circle A0 centre (-28.5, -24) radius 1.5
  circle A1 centre (28.5, 24) radius 1.5
  circle A2 centre (28.5, -24) radius 1.5
  circle A3 centre (-28.5, 24) radius 1.5
  line L0 (31.5, 27) -> (-31.5, 27)
  line L1 (-31.5, 27) -> (-31.5, -27)
  line L2 (-31.5, -27) -> (31.5, -27)
  line L3 (31.5, -27) -> (31.5, 27)
  line L4 (-15, -19.5) -> (15, -19.5)
  line L5 (12, -14.5) -> (-12, -14.5)
  circle A4 centre (14, -16.5) radius 1.5
  line L6 (15, -19.5) -> (17, -17.5)
  line L7 (17, -17.5) -> (17, 0)
  line L8 (17, 0) -> (12, 0)
  line L9 (12, 0) -> (12, -14.5)
  line L10 (-12, -14.5) -> (-12, 0)
  line L11 (-12, 0) -> (-17, 0)
  line L12 (-17, 0) -> (-17, -17.5)
  line L13 (-17, -17.5) -> (-15, -19.5)
  circle A5 centre (-14, -16.5) radius 1.5
  line L14 (12, 0) -> (-12, 0)
  line L15 (0, 0) -> (0, -7.25)
  line L16 (12, 0) -> (12, 14.5)
  line L17 (17, 17.5) -> (17, 0)
  line L18 (17, 0) -> (12, 0)
  line L19 (-15, 19.5) -> (15, 19.5)
  line L20 (12, 14.5) -> (-12, 14.5)
  line L21 (-12, 14.5) -> (-12, 0)
  circle A6 centre (14, 16.5) radius 1.5
  circle A7 centre (-14, 16.5) radius 1.5
  line L22 (-17, 17.5) -> (-15, 19.5)
  line L23 (-17, 0) -> (-17, 17.5)
  line L24 (-12, 0) -> (-17, 0)
  line L25 (15, 19.5) -> (17, 17.5)
  constraint perpendicular L10 L14
  constraint midpoint L14 L15.start
  constraint perpendicular L14 L15
  constraint symmetric L12.end L14 L22.start
  constraint symmetric L4.start L14 L19.start
  constraint symmetric L4.end L14 L19.end
  constraint symmetric L6.end L14 L17.start
  constraint symmetric L8.end L14 L9.start
  constraint symmetric L5.start L14 L16.end
  constraint symmetric L5.end L14 L20.end
  constraint symmetric L10.end L14 L11.start
  constraint symmetric L11.end L14 L12.start
  constraint symmetric L7.end L14 L8.start
  constraint symmetric A4 L14 A6
  constraint symmetric A5 L14 A7
extrude "Extrude2" add sketch "Sketch2" along normal blind 90 contours L4 L5 L6 L7 L8 L9 L10 L11 L12 L13 L18 L24 | L8 L11 L16 L17 L18 L19 L20 L21 L22 L23 L24 L25
fillet "Fillet1" radius 3 4 edges at (0, -27, 3) (-31.5, 0, 3) (31.5, 0, 3) (0, 27, 3)
sketch "Sketch3" plane through (0, 19.5, 0) normal (0, 1, 0) x (-1, 0, 0)
  line L0 (-15, 3) -> (15, 3)
  line L1 (15, 3) -> (15, 93)
  line L2 (15, 93) -> (-15, 93)
  line L3 (-15, 93) -> (-15, 3)
  line L4 (-15, 48) -> (15, 48)
  circle A0 centre (0, 48) radius 9.5
  dimension "d12" = 19
  constraint midpoint L3 L4.start
  constraint midpoint L1 L4.end
  constraint midpoint L4 A0.centre
  measures "d12" diameter of A0
extrude "Extrude3" cut sketch "Sketch3" against normal blind 6 contours L4 A0 | L4 A0
sketch "Sketch4" plane through (0, 0, 93) normal (0, 0, 1) x (-1, 0, 0)
  circle A0 centre (14, -16.5) radius 1.5
  circle A1 centre (14, 16.5) radius 1.5
  circle A2 centre (-14, -16.5) radius 1.5
  line L0 (12, 14.5) -> (12, -14.5)
  line L1 (12, -14.5) -> (-12, -14.5)
  line L2 (-12, -14.5) -> (-12, 14.5)
  line L3 (-12, 14.5) -> (12, 14.5)
  circle A3 centre (-14, 16.5) radius 1.5
  line L4 (-17, 17.5) -> (-17, -17.5)
  line L5 (-17, -17.5) -> (-15, -19.5)
  line L6 (-15, -19.5) -> (15, -19.5)
  line L7 (15, -19.5) -> (17, -17.5)
  line L8 (17, -17.5) -> (17, 17.5)
  line L9 (17, 17.5) -> (15, 19.5)
  line L10 (15, 19.5) -> (-15, 19.5)
  line L11 (-15, 19.5) -> (-17, 17.5)
  line L12 (-50, 0) -> (50, 0)
  line L13 (50, 0) -> (33.9234, 54.6299)
  line L14 (33.9234, 54.6299) -> (-46.2592, 44.9375)
  line L15 (-46.2592, 44.9375) -> (-50, 0)
  line L16 (12, 14.5) -> (-12, 14.5)
  line L17 (-12, 14.5) -> (-12, -14.5)
  line L18 (-12, -14.5) -> (12, -14.5)
  line L19 (12, -14.5) -> (12, 14.5)
  line L20 (-50, 0) -> (-64.2202, -68.1179)
  line L21 (-64.2202, -68.1179) -> (43.9074, -45.7813)
  line L22 (43.9074, -45.7813) -> (50, 0)
  constraint horizontal L12
extrude "Extrude4" cut sketch "Sketch4" against normal blind 500 contours A1 | L0 L2 L3 L4 L8 L9 L10 L11 L12 L16 L17 L19 | L0 L2 L3 L12 L16 L17 L19 | L0 L1 L2 L12 L17 L18 L19 | L4 L8 L9 L10 L11 L12 L13 L14 L15 | A3

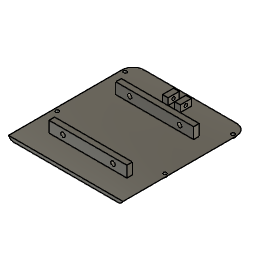
design "baseplate"
Autodesk Fusion 360 part; units mm, degrees
sketch "Sketch1" plane through (0, 0, 0) normal (0, 0, 1) x (1, 0, 0)
  line L0 (0, 0) -> (-51.5, 0)
  line L1 (0, 0) -> (51.5, 0)
  line L2 (-51.5, 0) -> (-51.5, 265)
  line L3 (-51.5, 265) -> (51.5, 265)
  line L4 (51.5, 265) -> (51.5, 0)
  dimension "d1" = 51.5
  dimension "d2" = 51.5
  dimension "d3" = 265
  constraint coincident L0.start L1.start
  constraint horizontal L0
  constraint parallel L0 L1
  constraint perpendicular L0 L2
  constraint perpendicular L2 L3
  constraint perpendicular L1 L4
  measures "d1" distance of L0.start L0.end
  measures "d2" distance of L0.start L1.end
  measures "d3" distance of L0.end L2.end
extrude "Extrude1" add sketch "Sketch1" along normal blind 3